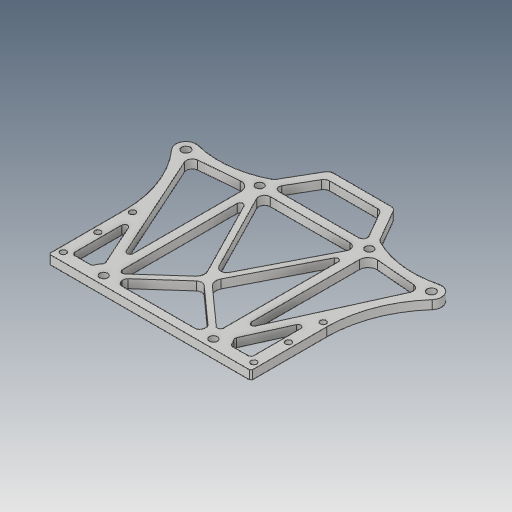
# Autodesk Inventor part: body_top_base_v1
Saved by Autodesk Inventor 2018 (Build 220112000, 112)
## iProperties
Created: 2018-08-31
Part Number: body_top_base_v1
Material: 一般
Document SubType Name: Modeling
Designer: student
Density: 1 g/cm^3
Appearance: 既定
Author: student
Autodesk Inventor part; units mm, degrees
ref_plane "YZ Plane" through (0, 0, 0) normal (1, 0, 0) x (0, 1, 0)
ref_plane "XZ Plane" through (0, 0, 0) normal (0, 1, 0) x (-1, 0, 0)
ref_plane "XY Plane" through (0, 0, 0) normal (0, 0, 1) x (1, 0, 0)
sketch "スケッチ1" plane through (0, 0, 0) normal (0, 1, 0) x (-1, 0, 0)
  circle A0 centre (-42.5, -35) radius 1.5
  line L0 (0, 0) -> (0, 1.3418)
  circle A1 centre (-19, -37) radius 1.4
  circle A2 centre (-19, 17) radius 1.4
  line L1 (-19, -37) -> (-19, 17) construction
  line L2 (0, -38.5) -> (0, -35.5)
  line L3 (-19, -37) -> (0, -37) construction
  line L4 (-19, -37) -> (-42.5, -35) construction
  line L5 (-42.5, -35) -> (-19, 17) construction
  line L6 (-19, 17) -> (0, 17) construction
  arc A3 (-18.7995, -40.9801) -> (-41.6304, -38.3902) centre (-33.6133, -69.644) ccw
  arc A4 (-45.1079, -32.6658) -> (-41.6304, -38.3902) centre (-42.5, -35) ccw
  line L7 (-23.7544, -35.0899) -> (-37.4424, -33.925)
  line L8 (-39.0953, -31.1086) -> (-22.4113, 5.8093)
  arc A5 (-39.0953, -31.1086) -> (-37.4424, -33.925) centre (-37.2728, -31.9322) ccw
  line L9 (-20.5, 5.3975) -> (-20.5, -32.1008)
  arc A6 (-23.7544, -35.0899) -> (-20.5, -32.1008) centre (-23.5, -32.1008) ccw
  arc A7 (-20.5, 5.3975) -> (-22.4113, 5.8093) centre (-21.5, 5.3975) ccw
  line L10 (-19, 17) -> (0, 0) construction
  line L11 (-19, -37) -> (0, 0) construction
  line L12 (-15.8332, 12.8247) -> (-2.9691, 1.3147)
  line L13 (-2.3008, -2.2914) -> (-15.6104, -28.2101)
  line L14 (-17.5, -27.7533) -> (-17.5, 12.0795)
  arc A8 (-15.8332, 12.8247) -> (-17.5, 12.0795) centre (-16.5, 12.0795) ccw
  arc A9 (-17.5, -27.7533) -> (-15.6104, -28.2101) centre (-16.5, -27.7533) ccw
  arc A10 (-2.3008, -2.2914) -> (-2.9691, 1.3147) centre (-4.9695, -0.921) ccw
  circle A11 centre (-19, 17) radius 3.5 construction
  line L15 (-42.8121, -36.4789) -> (-26.0599, -37.9046) construction
  line L16 (-33, 17) -> (-33, -7) construction
  circle A12 centre (-33, 17) radius 1.05
  circle A13 centre (-33, -7) radius 1.05
  circle A14 centre (-33, 5) radius 1.05
  line L17 (-34.5, 20) -> (0, 20)
  line L18 (0, 0) -> (24.0054, 0) construction
  line L19 (-35, -6.2168) -> (-35, 19.5)
  arc A15 (-45.1079, -32.6658) -> (-35, -6.2168) centre (-74.6579, -6.2168) ccw
  line L20 (-37.3423, -19.9448) -> (-34.4071, -13.45) construction
  line L21 (-33, 3.7852) -> (-33, 6.2148) construction
  line L22 (-22.6131, 12.6474) -> (-29.0887, -1.6817)
  line L23 (-31, -1.2698) -> (-31, 15)
  line L24 (-30, 16) -> (-24.6569, 16)
  arc A16 (-23.714, 15.3333) -> (-22.7703, 13.716) centre (-19, 17) ccw
  arc A17 (-31, -1.2698) -> (-29.0887, -1.6817) centre (-30, -1.2698) ccw
  arc A18 (-30, 16) -> (-31, 15) centre (-30, 15) ccw
  arc A19 (-23.714, 15.3333) -> (-24.6569, 16) centre (-24.6569, 15) ccw
  arc A20 (-22.6131, 12.6474) -> (-22.7703, 13.716) centre (-23.5244, 13.0592) ccw
  line L25 (-35, 19.5) -> (-34.5, 20)
  line L26 (-19, -37) -> (-10.3397, -52) construction
  line L27 (-10.3397, -52) -> (0, -52) construction
  arc A21 (-17.9857, -41.7568) -> (-18.7995, -40.9801) centre (-19.7178, -42.7568) ccw
  line L28 (-17.9857, -41.7568) -> (-11.7831, -52.5)
  line L29 (-10.0511, -53.5) -> (0, -53.5)
  line L30 (0, -53.5) -> (0, -50.5)
  line L31 (0, -50.5) -> (-8.319, -50.5)
  line L32 (-10.0511, -49.5) -> (-15.1029, -40.75)
  line L33 (-13.8038, -38.5) -> (0, -38.5)
  arc A22 (-13.8038, -38.5) -> (-15.1029, -40.75) centre (-13.8038, -40) ccw
  circle A23 centre (-19, -37) radius 3.5 construction
  arc A24 (-11.7831, -52.5) -> (-10.0511, -53.5) centre (-10.0511, -51.5) ccw
  arc A25 (-10.0511, -49.5) -> (-8.319, -50.5) centre (-8.319, -48.5) ccw
  line L34 (0, -35.5) -> (-13.8303, -35.5)
  line L35 (-15.6094, -32.5864) -> (0, -2.1891)
  arc A26 (-15.6094, -32.5864) -> (-13.8303, -35.5) centre (-13.8303, -33.5) ccw
  line L36 (0, -35.5) -> (0, -2.1891) construction
  line L37 (0, -2.1891) -> (0, 0)
  line L38 (0, 1.3418) -> (-13.8618, 13.7445)
  line L39 (-12.6754, 17) -> (0, 17)
  arc A27 (-14.2781, 15.3556) -> (-14.135, 15.8462) centre (-19, 17) ccw
  arc A28 (-14.2781, 15.3556) -> (-13.8618, 13.7445) centre (-12.8616, 14.8623) ccw
  arc A29 (-12.6754, 17) -> (-14.135, 15.8462) centre (-12.6754, 15.5) ccw
  line L40 (0, 1.3418) -> (0, 17) construction
  line L41 (0, 17) -> (0, 20)
  point P0 (-19, -10)
  point P1 (-1.2424, -0.2302)
  point P2 (-22.3312, 13.2713)
  point P3 (-23.899, 16)
  point P4 (-35, 20)
  point P5 (-14.6823, 14.4786)
  point P6 (-14, 17)
  dimension "d2" = 38
  dimension "d3" = 54
  dimension "d4" = 2.8
  dimension "d17" = 1.5
  dimension "d18" = 3
  dimension "d19" = 1
  dimension "d21" = 3
  dimension "d22" = 1
  dimension "d23" = 3
  dimension "d34" = 2.1
  dimension "d47" = 3
  dimension "d49" = 85
  dimension "d51" = 35
  dimension "d55" = 24
  dimension "d60" = 2
  dimension "d61" = 3
  dimension "d63" = 2
  dimension "d64" = 4
  dimension "d65" = 1.5
  dimension "d66" = 5
  dimension "d67" = 1
  dimension "d68" = 0.5
  dimension "d69" = 0.5
  dimension "d70" = 70
  dimension "d71" = 2
  dimension "d72" = 1.5
  dimension "d73" = 3.5
  dimension "d74" = 1.5
  dimension "d75" = 2
  dimension "d76" = 7
  dimension "d77" = 60
  dimension "d78" = 3
  dimension "d79" = 3
  dimension "d80" = 15
  dimension "d82" = 2
  dimension "d83" = 2
  dimension "d84" = 3
  dimension "d85" = 2
  dimension "d86" = 1
  dimension "d87" = 1.5
  dimension "d88" = 3
  dimension "d90" = 2
  dimension "d91" = 5
  dimension "d93" = 2
  constraints: 84 end point, 48 point on circle, 40 tangent, 30 centre point, 12 point on line, 10 parallel, 10 vertical, 9 equal radius, 8 horizontal, 8 perpendicular, 5 coincident, 5 midpoint, 3 collinear, 3 concentric, 1 horizontal alignment, 7 other
  measures "d2" diameter of L1 L0
  measures "d3" distance of L1.start L1.end
  measures "d4" diameter of A1
  measures "d17" distance between parallel lines of L7 L4
  measures "d18" radius of A6
  measures "d19" radius of A7
  measures "d21" distance between parallel lines of L14 L9
  measures "d22" radius of A8
  measures "d23" radius of A10
  measures "d34" diameter of A13
  measures "d47" distance from line of L17 A12.centre
  measures "d49" diameter of L4.end L2
  measures "d51" distance from line of L18 L4.end
  measures "d55" distance of L16.start L16.end
  measures "d60" radius of A5
  measures "d61" diameter of A0
  measures "d63" distance from line of L23 A14.centre
  measures "d64" distance between parallel lines of L17 L24
  measures "d65" distance between parallel lines of L5 L22
  measures "d66" radius of A16
  measures "d67" radius of A17
  measures "d68" distance of L19.end point (-35, 20)
  measures "d69" distance of L17.start point (-35, 20)
  measures "d70" diameter of L19 L0
  measures "d71" distance between parallel lines of L19 L16
  measures "d72" distance between parallel lines of L5 L20
  measures "d73" radius of A4
  measures "d74" radius of A22
  measures "d75" radius of A21
  measures "d76" diameter of A23
  measures "d77" angle of L3 L26
  measures "d78" distance between parallel lines of L28 L32
  measures "d79" distance between parallel lines of L29 L31
  measures "d80" distance between parallel lines of L3 L27
  measures "d82" radius of A24
  measures "d83" radius of A26
  measures "d84" distance between parallel lines of L34 L33
  measures "d85" distance between parallel lines of L35 L13
  measures "d86" radius of A9
  measures "d87" radius of A28
  measures "d88" distance between parallel lines of L17 L39
  measures "d90" distance between parallel lines of L38 L12
  measures "d91" radius of A27
  measures "d93" distance from line of L4.end L3
extrude "押し出し1" add sketch "スケッチ1" along normal blind 3
mirror "ミラー1" about plane through (0, 0, 0) normal (1, 0, 0) of "押し出し1"
fillet "フィレット1" radius 2 2 edges at (0, 1.5, -2.1891) (0, 1.5, 1.3418)
